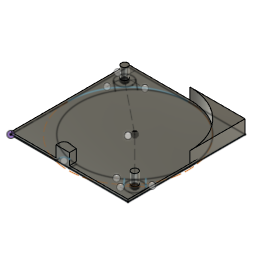
5015_TestBench v2 (Autodesk Fusion 360 design; units mm, degrees)
Autodesk Fusion 360 part; units mm, degrees
sketch "Sketch1" plane through (0, 0, 0) normal (0, 0, 1) x (1, 0, 0)
  line L0 (0, 0) -> (52, 0)
  line L1 (52, 0) -> (52, 52)
  line L2 (52, 52) -> (0, 52)
  line L3 (0, 52) -> (0, 0)
  circle A0 centre (27.5, 27.5) radius 24.5
  line L4 (0, 0) -> (0, 25) construction
  arc A1 (0, 25.4649) -> (26.5351, 52) centre (26.5351, 25.4649) ccw construction
  arc A2 (26.5351, 52) -> (0, 25.4649) centre (26.5351, 25.4649) ccw
  line L5 (0, 0) -> (20, 0)
  line L6 (20, 0) -> (20, 0.4966)
  line L7 (20, 0.4966) -> (20, 1.5703)
  line L8 (22.5173, 3.5022) -> (22.3423, 3.549)
  arc A3 (22.5173, 3.5022) -> (20, 1.5703) centre (22, 1.5703) ccw
  line L9 (3, 52) -> (3, 39.6785) construction
  line L10 (0, 47.5) -> (12.0217, 47.5) construction
  circle A4 centre (4.5, 46) radius 1.5
  circle A5 centre (4.5, 46) radius 3.5
  line L11 (51, 0) -> (51, 11.6338) construction
  line L12 (52, 4) -> (44.6522, 4) construction
  circle A6 centre (47.5, 7.5) radius 3.5
  circle A7 centre (47.5, 7.5) radius 1.5
  line L13 (40.311, 6.6239) -> (40.2361, 6.5706) construction
  line L14 (27.5, 27.5) -> (47.5, 7.5) construction
  line L15 (47.5, 7.5) -> (44.8851, 5.1736) construction
  line L16 (47.5, 7.5) -> (50.1149, 9.8264) construction
  line L17 (50.1149, 9.8264) -> (47.1177, 12.8236)
  line L18 (44.8851, 5.1736) -> (42.3551, 8.0173)
  line L19 (27.5, 27.5) -> (4.5, 46) construction
  line L20 (4.5, 46) -> (6.6937, 48.7272) construction
  line L21 (4.5, 46) -> (2.3063, 43.2728) construction
  line L22 (2.3063, 43.2728) -> (6.4114, 39.9708)
  line L23 (6.6937, 48.7272) -> (10.7987, 45.4253)
  line L24 (26, 0) -> (26, 3.046)
  dimension "d34" = 52
  dimension "d35" = 52
  dimension "d36" = 24.5
  dimension "d37" = 25
  dimension "d38" = 20
  dimension "d39" = 2
  dimension "d40" = 3
  dimension "d41" = 4.5
  dimension "d42" = 1.5
  dimension "d43" = 7
  dimension "d46" = 1
  dimension "d48" = 4
  dimension "d49" = 3.5
  dimension "d50" = 3
  constraint horizontal L0
  constraint vertical L1
  constraint horizontal L2
  constraint vertical L3
  constraint coincident L0.start L3.end
  constraint tangent L2 A0
  constraint tangent L1 A0
  constraint coincident L3 L4.end
  constraint tangent L2 A1
  constraint tangent L3 A1
  constraint coincident L2 A1.end
  constraint coincident L3 A1.start
  constraint concentric A1 A2
  constraint coincident L0 L5.end
  constraint perpendicular L5 L6
  constraint perpendicular L5 L7
  constraint coincident A0 L8.end
  constraint tangent L8 A3
  constraint tangent L7 A3
  constraint coincident L2 L9.start
  constraint perpendicular L2 L9
  constraint horizontal L10
  constraint tangent L10 A4
  constraint tangent L9 A4
  constraint concentric A4 A5
  constraint coincident L0 L11.start
  constraint perpendicular L0 L11
  constraint coincident L1 L12.start
  constraint perpendicular L11 L12
  constraint tangent L12 A6
  constraint tangent L11 A6
  constraint concentric A6 A7
  constraint coincident A6 L15.end
  constraint coincident A0 L13.end
  constraint coincident A0.centre L14.start
  constraint coincident A6.centre A7.centre
  constraint coincident A6 L16.end
  constraint parallel L15 L16
  constraint coincident A0 L17.end
  constraint parallel L14 L17
  constraint coincident A0 L18.end
  constraint tangent A6 L18
  constraint coincident A4.centre A5.centre
  constraint coincident A5 L20.end
  constraint perpendicular L19 L20
  constraint coincident A5 L21.end
  constraint parallel L20 L21
  constraint coincident A0 L22.end
  constraint tangent A5 L22
  constraint coincident A0 L23.end
  constraint tangent A5 L23
  constraint midpoint L0 L24.start
  constraint coincident A0 L24.end
  constraint perpendicular L0 L24
  measures "d34" distance of L0.start L0.end
  measures "d35" distance of L0.start L2.end
  measures "d36" radius of A0
  measures "d37" distance of L0.start L4.end
  measures "d38" distance of L0.start L5.end
  measures "d39" radius of A3
  measures "d40" distance of L3 L9
  measures "d41" distance of L2 L10
  measures "d42" radius of A4
  measures "d43" diameter of A5
  measures "d46" distance of L1 L11
  measures "d48" distance of L0 L12
  measures "d49" radius of A6
  measures "d50" diameter of A7
extrude "Extrude8" add sketch "Sketch1" along normal blind 1 contours L0 L3 A0 A2 L5 L6 L7 L8 A3 L22 | L2 L3 A2 A5 L22 L23 | L0 L1 A0 A6 L17 L18 L24 | A2 A5 L22 L23 | A0 A2 L22 L23 | A0 | L2 A0 A2 L23 | A5 | A0 A6 L17 L18 | A6 L17 picked at (49.7596, 9.1981)
extrude "Extrude9" add sketch "Sketch1" along normal blind 6 contours L0 A0 L6 L7 L8 A3 L24 | L1 L2 A0 | A4 | A7
